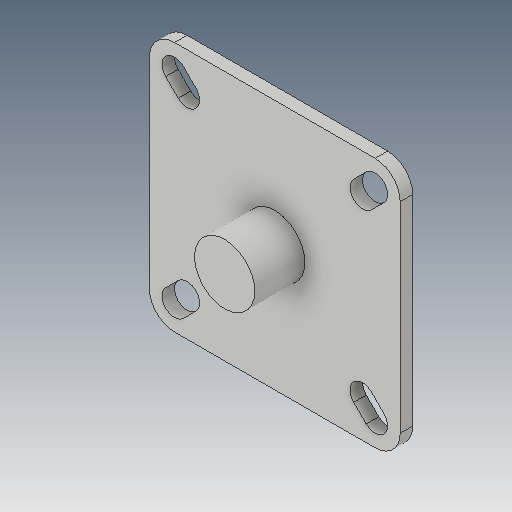
# Autodesk Inventor part: 自由輪パーツ2
Saved by Autodesk Inventor 2020.3 (Build 243373000, 373)
## iProperties
Part Number: 自由輪パーツ2
Material: 一般
Document SubType Name: Modeling
Designer: highs
Density: 1 g/cm^3
Appearance: 既定
Description: https://www.monotaro.com/p/3519/5946/
Stock Number: ナンシン プレート式 自在、ゴム(B入り)車 車輪径D 150Φmm、許容荷重 160daN、STC-150CBC
Author: highs
Autodesk Inventor part; units mm, degrees
ref_plane "YZ Plane" through (0, 0, 0) normal (1, 0, 0) x (0, 1, 0)
ref_plane "XZ Plane" through (0, 0, 0) normal (0, 1, 0) x (-1, 0, 0)
ref_plane "XY Plane" through (0, 0, 0) normal (0, 0, 1) x (1, 0, 0)
sketch "スケッチ1" plane through (0, 0, 0) normal (0, 0, 1) x (1, 0, 0)
  line L0 (-50, -50) -> (50, -50)
  line L1 (50, -50) -> (50, 50)
  line L2 (50, 50) -> (-50, 50)
  line L3 (-50, 50) -> (-50, -50)
  line L4 (-50, -50) -> (50, 50) construction
  line L5 (50, -50) -> (-50, 50) construction
  line L6 (35, 35) -> (40, 40) construction
  line L7 (31.4645, 38.5355) -> (36.4645, 43.5355)
  line L8 (43.5355, 36.4645) -> (38.5355, 31.4645)
  arc A0 (31.4645, 38.5355) -> (38.5355, 31.4645) centre (35, 35) ccw
  arc A1 (43.5355, 36.4645) -> (36.4645, 43.5355) centre (40, 40) ccw
  line L9 (-50, 0) -> (50, 0) construction
  line L10 (0, 50) -> (0, -50) construction
  line L11 (-35, 35) -> (-40, 40) construction
  line L12 (-31.4645, 38.5355) -> (-36.4645, 43.5355)
  line L13 (-43.5355, 36.4645) -> (-38.5355, 31.4645)
  arc A2 (-38.5355, 31.4645) -> (-31.4645, 38.5355) centre (-35, 35) ccw
  arc A3 (-36.4645, 43.5355) -> (-43.5355, 36.4645) centre (-40, 40) ccw
  line L14 (35, -35) -> (40, -40) construction
  line L15 (31.4645, -38.5355) -> (36.4645, -43.5355)
  line L16 (43.5355, -36.4645) -> (38.5355, -31.4645)
  arc A4 (38.5355, -31.4645) -> (31.4645, -38.5355) centre (35, -35) ccw
  arc A5 (36.4645, -43.5355) -> (43.5355, -36.4645) centre (40, -40) ccw
  arc A6 (-31.4645, -38.5355) -> (-38.5355, -31.4645) centre (-35, -35) ccw
  line L17 (-43.5355, -36.4645) -> (-38.5355, -31.4645)
  line L18 (-35, -35) -> (-40, -40) construction
  arc A7 (-43.5355, -36.4645) -> (-36.4645, -43.5355) centre (-40, -40) ccw
  line L19 (-31.4645, -38.5355) -> (-36.4645, -43.5355)
  point P0 (0, 0)
  point P1 (37.5, 37.5)
  point P2 (-37.5, 37.5)
  point P3 (37.5, -37.5)
  point P4 (-37.5, -37.5)
  dimension "d0" = 100
  dimension "d1" = 100
  dimension "d2" = 10
  dimension "d3" = 15
  dimension "d4" = 5
  constraints: 48 end point, 21 symmetric about line, 16 point on circle, 8 centre point, 7 midpoint, 4 tangent, 3 parallel, 2 point on line, 1 horizontal, 1 perpendicular, 6 other
  measures "d0" distance of L0.end L1.end
  measures "d1" distance between parallel lines of L1 L3
  measures "d2" distance from line of L2 L6.end
  measures "d3" distance from line of L2 L6.start
  measures "d4" radius of A1
extrude "押し出し1" add sketch "スケッチ1" along normal blind 5
fillet "フィレット1" radius 10 4 edges at (50, 50, 2.5) (50, -50, 2.5) (-50, -50, 2.5) (-50, 50, 2.5)
sketch "スケッチ2" plane through (0, 0, 5) normal (0, 0, 1) x (1, 0, 0)
  circle A0 centre (0, 0) radius 12
  dimension "d8" = 24
  constraints: 1 centre point, 1 coincident
  measures "d8" diameter of A0
extrude "押し出し2" add sketch "スケッチ2" along normal blind 20
